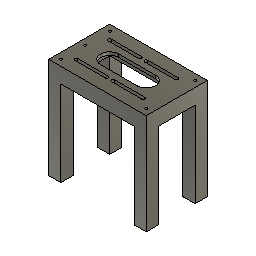
Direction_Motor_Mount (Autodesk Fusion 360 design; units mm, degrees)
Autodesk Fusion 360 part; units mm, degrees
ref_plane "WorkPlane1" through (0, 160, 0) normal (0, 1, 0) x (0, 0, 1)
sketch "Sketch1" plane through (0, 160, 0) normal (0, 1, 0) x (1, 0, 0)
  line L0 (80, 50) -> (-80, 50)
  line L1 (-80, 50) -> (-80, -50)
  line L2 (-80, -50) -> (80, -50)
  line L3 (80, -50) -> (80, 50)
  line L4 (80, 50) -> (-80, -50) construction
  line L5 (-80, 50) -> (80, -50) construction
  line L6 (-60, -30) -> (60, -30)
  line L7 (60, -30) -> (60, 30) construction
  line L8 (60, 30) -> (-60, 30) construction
  line L9 (-60, 30) -> (-60, -30) construction
  line L10 (-60, 0) -> (60, 0) construction
  line L11 (-30, 15) -> (30, 15)
  line L12 (30, -15) -> (-30, -15)
  arc A0 (-30, 15) -> (-30, -15) centre (-30, 0) ccw
  arc A1 (30, -15) -> (30, 15) centre (30, 0) ccw
  circle A2 centre (-57.5, 27.5) radius 2.5
  line L13 (0, 30) -> (0, -30) construction
  circle A3 centre (-2.5, 27.5) radius 2.5 construction
  circle A4 centre (-2.5, -27.5) radius 2.5 construction
  circle A5 centre (-57.5, -27.5) radius 2.5
  line L14 (-57.5, 27.5) -> (-2.5, -27.5) construction
  line L15 (-2.5, 27.5) -> (-57.5, -27.5) construction
  circle A6 centre (2.5, 27.5) radius 2.5
  circle A7 centre (57.5, 27.5) radius 2.5 construction
  circle A8 centre (57.5, -27.5) radius 2.5 construction
  circle A9 centre (2.5, -27.5) radius 2.5
  circle A10 centre (-7.5, -27.5) radius 2.5
  circle A11 centre (-7.5, 27.5) radius 2.5
  circle A12 centre (52.5, 27.5) radius 2.5
  circle A13 centre (52.5, -27.5) radius 2.5
  line L16 (-57.5, -25) -> (-7.5, -25)
  line L17 (-7.5, -30) -> (-57.5, -30)
  line L18 (2.5, -25) -> (52.5, -25)
  line L19 (52.5, -30) -> (2.5, -30)
  line L20 (-60, 30) -> (60, 30)
  line L21 (-57.5, 25) -> (-7.5, 25)
  line L22 (2.5, 25) -> (52.5, 25)
  line L23 (-60, -30) -> (-80, -50) construction
  line L24 (-60, 30) -> (-80, 50) construction
  line L25 (60, 30) -> (80, 50) construction
  line L26 (60, -30) -> (80, -50) construction
  line L27 (-70, 40) -> (-70, -40) construction
  circle A14 centre (-70, 0) radius 2
  circle A15 centre (-70, 40) radius 2
  circle A16 centre (-70, -40) radius 2
  circle A17 centre (70, -40) radius 2
  circle A18 centre (70, 40) radius 2
  point P0 (30, 0)
  dimension "d2" = 160
  dimension "d3" = 100
  dimension "d4" = -20
  dimension "d5" = 30
  dimension "d6" = 30
  dimension "d7" = 30
  dimension "d8" = 30
  dimension "d9" = 5
  dimension "d10" = 5
  dimension "d11" = 5
  dimension "d12" = 5
  dimension "d13" = 5
  dimension "d16" = 4
  dimension "d17" = 4
  dimension "d18" = 4
  dimension "d19" = 4
  dimension "d20" = 4
  constraint horizontal L0
  constraint perpendicular L0 L1
  constraint parallel L0 L2
  constraint parallel L1 L3
  constraint coincident L4 origin
  constraint coincident L5 origin
  constraint midpoint L9 L10.start
  constraint midpoint L7 L10.end
  constraint coincident P0 L10
  constraint coincident A0.centre L10
  constraint tangent L11 A0
  constraint horizontal L11
  constraint tangent L12 A0
  constraint parallel L11 L12
  constraint tangent L8 A2
  constraint tangent L9 A2
  constraint midpoint L8 L13.start
  constraint midpoint L6 L13.end
  constraint tangent L8 A3
  constraint tangent L13 A3
  constraint symmetric L10 A2 A5
  constraint symmetric L10 A3 A4
  constraint coincident A2.centre L14.start
  constraint coincident A4.centre L14.end
  constraint coincident A3.centre L15.start
  constraint coincident A5.centre L15.end
  constraint symmetric A0.centre L13 P0
  constraint symmetric A2 L13 A7
  constraint symmetric L13 A3 A6
  constraint symmetric L13 A4 A9
  constraint symmetric L13 A5 A8
  constraint tangent L6 A10
  constraint tangent A4 A10
  constraint symmetric L10 A10 A11
  constraint tangent L8 A12
  constraint tangent A7 A12
  constraint tangent L6 A13
  constraint tangent A8 A13
  constraint coincident A5 L16.start
  constraint coincident A10 L16.end
  constraint tangent A10 L16
  constraint coincident A10 L17.start
  constraint coincident A5 L17.end
  constraint coincident L6 L17.end
  constraint tangent A5 L17
  constraint coincident A9 L18.start
  constraint coincident A13 L18.end
  constraint tangent A13 L18
  constraint coincident A13 L19.start
  constraint coincident A9 L19.end
  constraint coincident L6 L19.end
  constraint tangent A9 L19
  constraint tangent A5 L16
  constraint tangent A9 L18
  constraint symmetric L6.start L10 L8.end
  constraint symmetric L6.end L10 L7.end
  constraint symmetric L10 L16.start L21.start
  constraint symmetric L10 L16.end L21.end
  constraint symmetric L10 L18.start L22.start
  constraint symmetric L10 L18.end L22.end
  constraint midpoint L24 L27.start
  constraint midpoint L23 L27.end
  constraint midpoint L27 A14.centre
  constraint coincident L27.start A15.centre
  constraint coincident L27.end A16.centre
  constraint midpoint L26 A17.centre
  constraint midpoint L25 A18.centre
  measures "d2" distance of L1.end L2.end
  measures "d3" distance of L0.end L1.end
  measures "d5" diameter of A0
  measures "d6" diameter of A1
  measures "d7" distance of L9 A0.centre
  measures "d8" distance of L7 P0
  measures "d9" diameter of A2
  measures "d10" diameter of A3
  measures "d11" diameter of A10
  measures "d12" diameter of A13
  measures "d13" diameter of A12
  measures "d16" diameter of A14
  measures "d17" diameter of A15
  measures "d18" diameter of A16
  measures "d19" diameter of A17
  measures "d20" diameter of A18
extrude "Extrude1" add sketch "Sketch1" along normal blind 5
sketch "Sketch2" plane through (0, 160, 0) normal (0, -1, 0) x (1, 0, 0)
  circle A0 centre (70, -40) radius 2
  circle A1 centre (70, 40) radius 2
  circle A2 centre (-70, 0) radius 2
  circle A3 centre (-70, -40) radius 2
  circle A4 centre (-70, 40) radius 2
  arc A5 (-57.5, -25) -> (-57.5, -30) centre (-57.5, -27.5) ccw
  line L0 (-57.5, -25) -> (-7.5, -25)
  arc A6 (-7.5, -30) -> (-7.5, -25) centre (-7.5, -27.5) ccw
  line L1 (-7.5, -30) -> (-57.5, -30)
  arc A7 (2.5, -25) -> (2.5, -30) centre (2.5, -27.5) ccw
  line L2 (2.5, -25) -> (52.5, -25)
  arc A8 (52.5, -30) -> (52.5, -25) centre (52.5, -27.5) ccw
  line L3 (52.5, -30) -> (2.5, -30)
  arc A9 (-30, 15) -> (-30, -15) centre (-30, 0) ccw
  line L4 (-30, 15) -> (30, 15)
  arc A10 (30, -15) -> (30, 15) centre (30, 0) ccw
  line L5 (30, -15) -> (-30, -15)
  arc A11 (-57.5, 30) -> (-57.5, 25) centre (-57.5, 27.5) ccw
  line L6 (-57.5, 30) -> (-7.5, 30)
  arc A12 (-7.5, 25) -> (-7.5, 30) centre (-7.5, 27.5) ccw
  line L7 (-7.5, 25) -> (-57.5, 25)
  arc A13 (2.5, 30) -> (2.5, 25) centre (2.5, 27.5) ccw
  line L8 (2.5, 30) -> (52.5, 30)
  arc A14 (52.5, 25) -> (52.5, 30) centre (52.5, 27.5) ccw
  line L9 (52.5, 25) -> (2.5, 25)
  line L10 (80, -50) -> (80, 50)
  line L11 (80, 50) -> (-80, 50)
  line L12 (-80, 50) -> (-80, -50)
  line L13 (-80, -50) -> (80, -50)
  line L14 (-80, -50) -> (80, -50)
  line L15 (80, -50) -> (80, -30)
  line L16 (80, -30) -> (-80, -30)
  line L17 (-80, -30) -> (-80, -50)
  line L18 (1.75, 0) -> (22.5, 0)
  line L19 (-80, 50) -> (80, 50)
  line L20 (80, 50) -> (80, 30)
  line L21 (80, 30) -> (-80, 30)
  line L22 (-80, 30) -> (-80, 50)
  line L23 (-80, 30) -> (-60, 30)
  line L24 (-60, 30) -> (-60, -30)
  line L25 (-60, -30) -> (-80, -30)
  line L26 (-80, -30) -> (-80, 30)
  line L27 (0, 1.75) -> (0, 22.5)
  line L28 (80, 30) -> (60, 30)
  line L29 (60, 30) -> (60, -30)
  line L30 (60, -30) -> (80, -30)
  line L31 (80, -30) -> (80, 30)
  dimension "d21" = 20
  dimension "d22" = 20
  dimension "d23" = 60
  constraint horizontal L14
  constraint vertical L15
  constraint horizontal L16
  constraint vertical L17
  constraint coincident L12.end L13.start
  constraint symmetric L12.end L18 L11.end
  constraint symmetric L10.start L18 L10.end
  constraint symmetric L15.end L18 L20.end
  constraint symmetric L16.end L18 L21.end
  constraint horizontal L23
  constraint vertical L24
  constraint horizontal L25
  constraint vertical L26
  constraint symmetric L21.end L27 L20.end
  constraint symmetric L23.end L27 L28.end
  constraint symmetric L24.end L27 L29.end
  constraint symmetric L16.end L27 L15.end
  measures "d21" distance of L12.end L16.end
  measures "d22" distance of L21.end L23.end
  measures "d23" distance of L21.end L16.end
extrude "Extrude2" add sketch "Sketch2" along normal blind 20 contours A0 | A1 | A2 | A3 | A4 | L12 L16 L21 L23 L24 L25 L26 | L1 L3 L10 L12 L13 L14 L15 L16 L17 L25 L30 | L6 L8 L10 L11 L12 L19 L20 L21 L22 L23 L28 | L10 L16 L21 L28 L29 L30 L31
sketch "Sketch3" plane through (0, 140, 0) normal (0, -1, 0) x (1, 0, 0)
  line L0 (-60, 30) -> (60, 30)
  line L1 (60, 30) -> (60, -30)
  line L2 (60, -30) -> (-60, -30)
  line L3 (-60, -30) -> (-60, 30)
  line L4 (-80, 50) -> (-80, -50)
  line L5 (-80, -50) -> (80, -50)
  line L6 (80, -50) -> (80, 50)
  line L7 (80, 50) -> (-80, 50)
  line L8 (-80, 50) -> (-60, 50)
  line L9 (-60, 50) -> (-60, 30)
  line L10 (-60, 30) -> (-80, 30)
  line L11 (-80, 30) -> (-80, 50)
  line L12 (60, 30) -> (80, 30)
  line L13 (80, 30) -> (80, 50)
  line L14 (80, 50) -> (60, 50)
  line L15 (60, 50) -> (60, 30)
  line L16 (60, -30) -> (80, -30)
  line L17 (80, -30) -> (80, -50)
  line L18 (80, -50) -> (60, -50)
  line L19 (60, -50) -> (60, -30)
  line L20 (-60, -30) -> (-80, -30)
  line L21 (-80, -30) -> (-80, -50)
  line L22 (-80, -50) -> (-60, -50)
  line L23 (-60, -50) -> (-60, -30)
  constraint horizontal L8
  constraint vertical L9
  constraint horizontal L10
  constraint vertical L11
  constraint coincident L0.start L3.end
  constraint coincident L4.start L7.end
  constraint horizontal L12
  constraint vertical L13
  constraint horizontal L14
  constraint vertical L15
  constraint coincident L6.end L7.start
  constraint coincident L0.end L1.start
  constraint horizontal L16
  constraint vertical L17
  constraint horizontal L18
  constraint vertical L19
  constraint coincident L5.end L6.start
  constraint coincident L1.end L2.start
  constraint horizontal L20
  constraint vertical L21
  constraint horizontal L22
  constraint vertical L23
  constraint coincident L4.end L5.start
  constraint coincident L2.end L3.start
extrude "Extrude3" add sketch "Sketch3" along normal blind 140 contours L4 L7 L8 L9 L10 L11 | L6 L7 L12 L13 L14 L15 | L4 L5 L20 L21 L22 L23 | L5 L6 L16 L17 L18 L19
sketch "Sketch4" plane through (-80, 0, 0) normal (-1, 0, 0) x (0, 0, 1)
  line L0 (50, 0) -> (50, 165)
  line L1 (50, 165) -> (-50, 165)
  line L2 (-50, 165) -> (-50, 0)
  line L3 (-50, 0) -> (-30, 0)
  line L4 (-30, 0) -> (-30, 140)
  line L5 (-30, 140) -> (30, 140)
  line L6 (30, 140) -> (30, 0)
  line L7 (30, 0) -> (50, 0)
  line L8 (0, 165) -> (0, 140) construction
  circle A0 centre (0, 152.5) radius 5
  dimension "d28" = 10
  constraint midpoint L1 L8.start
  constraint midpoint L5 L8.end
  constraint midpoint L8 A0.centre
  measures "d28" diameter of A0
extrude "Extrude4" cut sketch "Sketch4" against normal up to surface (20 mm away) contours A0
move_body "Move1" bodies 1 to x (1, 0, 0) y (0, 0, 1) z (0, -1, 0) at (0, 0, 0)
scale "Scale1" factor 0.1 about (0, 0, 0) bodies 1
scale "Scale2" factor 0.01 about (0, 0, 0) bodies 1
equation "d8 = d7"
equation "d10 = d9"
equation "d11 = d9"
equation "d12 = d11"
equation "d13 = d12"
